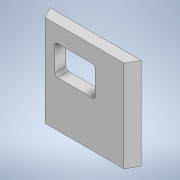
# Autodesk Inventor part: SatelliteSideWallCamera_v2
Saved by Autodesk Inventor 2020 (Build 240168000, 168)
## iProperties
Created: 2020-03-05
Part Number: SatelliteSideWallCamera_v2
Material: Generic
Document SubType Name: Modeling
Designer: WANG
Density: 1 g/cm^3
Appearance: Default
Author: WANG
Autodesk Inventor part; units mm, degrees
ref_plane "YZ Plane" through (0, 0, 0) normal (1, 0, 0) x (0, 1, 0)
ref_plane "XZ Plane" through (0, 0, 0) normal (0, 1, 0) x (-1, 0, 0)
ref_plane "XY Plane" through (0, 0, 0) normal (0, 0, 1) x (1, 0, 0)
sketch "Sketch1" plane through (0, 0, 0) normal (0, 1, 0) x (-1, 0, 0)
  line L0 (-107.95, -0.0035) -> (-53.978, 93.4857)
  line L1 (-53.978, 93.4857) -> (53.972, 93.4892)
  line L2 (53.972, 93.4892) -> (107.95, 0.0035)
  line L3 (107.95, 0.0035) -> (53.978, -93.4857)
  line L4 (53.978, -93.4857) -> (-53.972, -93.4892)
  line L5 (-53.972, -93.4892) -> (-107.95, -0.0035)
  line L6 (-92.964, 0.0336) -> (-46.4529, 80.526)
  line L7 (-46.4529, 80.526) -> (46.5111, 80.4924)
  line L8 (46.5111, 80.4924) -> (92.964, -0.0336)
  line L9 (92.964, -0.0336) -> (46.4529, -80.526)
  line L10 (46.4529, -80.526) -> (-46.5111, -80.4924)
  line L11 (-46.5111, -80.4924) -> (-92.964, 0.0336)
  line L12 (53.978, -93.4857) -> (46.4529, -80.526)
  line L13 (-53.972, -93.4892) -> (-46.5111, -80.4924)
  point P0 (0, 0)
  point P1 (0, 0)
  point P2 (0, 0)
  point P3 (0, 0)
  dimension "d0" = 215.9
  dimension "d1" = 14.986
  constraints: 28 end point, 2 coincident, 26 other
  measures "d0" distance of L0.start L2.end
  measures "d1" distance of L0.start L6.start
extrude "Extrusion1" add sketch "Sketch1" along normal blind 107.95 contours L13 L10 L12 L4
sketch "Sketch2" plane through (53.972, 0, -93.4892) normal (0, 0, -1) x (-1, 0, 0)
  line L0 (85.725, 88.9) -> (44.45, 88.9)
  line L1 (41.275, 85.725) -> (41.275, 57.15)
  line L2 (44.45, 53.975) -> (85.725, 53.975)
  line L3 (88.9, 57.15) -> (88.9, 85.725)
  line L4 (107.95, 0) -> (107.95, 107.95) projected
  line L5 (0, 107.95) -> (107.95, 107.95) projected
  arc A0 (44.45, 88.9) -> (41.275, 85.725) centre (44.45, 85.725) ccw
  arc A1 (88.9, 85.725) -> (85.725, 88.9) centre (85.725, 85.725) ccw
  arc A2 (41.275, 57.15) -> (44.45, 53.975) centre (44.45, 57.15) ccw
  arc A3 (85.725, 53.975) -> (88.9, 57.15) centre (85.725, 57.15) ccw
  point P0 (53.975, 0)
  point P1 (41.275, 53.975)
  point P2 (41.275, 88.9)
  point P3 (88.9, 53.975)
  dimension "d4" = 47.625
  dimension "d5" = 34.925
  dimension "d6" = 19.05
  dimension "d7" = 19.05
  dimension "d8" = 3.175
  constraints: 8 end point, 8 point on circle, 8 tangent, 6 point on line, 4 centre point, 3 equal radius, 2 parallel, 1 horizontal, 1 perpendicular
  measures "d4" distance of point (88.9, 53.975) point (41.275, 53.975)
  measures "d5" distance of point (41.275, 53.975) point (41.275, 88.9)
  measures "d6" distance between parallel lines of L4 L3
  measures "d7" distance between parallel lines of L5 L0
  measures "d8" radius of A0
extrude "Extrusion2" cut sketch "Sketch2" against normal up to surface (12.9994 mm away)
body "Solid1"
